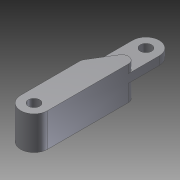
# Autodesk Inventor part: F
Saved by Autodesk Inventor 2011 SP2 (Build 150309200, 309)
## iProperties
Created: 2014-05-09
Part Number: F
Document SubType Name: Modeling
Designer: Maurice Woods
Density: 1 g/cm^3
Author: Maurice Woods
Autodesk Inventor part; units mm, degrees
ref_plane "YZ Plane" through (0, 0, 0) normal (1, 0, 0) x (0, 1, 0)
ref_plane "XZ Plane" through (0, 0, 0) normal (0, 1, 0) x (-1, 0, 0)
ref_plane "XY Plane" through (0, 0, 0) normal (0, 0, 1) x (1, 0, 0)
sketch "Sketch1" plane through (0, 0, 0) normal (0, 0, 1) x (1, 0, 0)
  line L0 (0, 20.7105) -> (0, 20.7105)
  line L1 (4, 16.7105) -> (4, 14.6095)
  line L2 (0, -20.7105) -> (0, -20.7105)
  line L3 (-4, -16.7105) -> (-4, 1.4635)
  line L4 (-4, 20.7105) -> (0, 20.7105) construction
  line L5 (0, 20.7105) -> (0, 0) construction
  line L6 (0, 0) -> (-4, 0) construction
  line L7 (-4, 0) -> (-4, 20.7105) construction
  arc A0 (4, 16.7105) -> (0, 20.7105) centre (0, 16.7105) ccw
  arc A1 (0, 20.7105) -> (-4, 16.7105) centre (0, 16.7105) ccw
  arc A2 (-4, -16.7105) -> (0, -20.7105) centre (0, -16.7105) ccw
  arc A3 (0, -20.7105) -> (4, -16.7105) centre (0, -16.7105) ccw
  line L8 (-4, 1.4635) -> (4, 14.6095)
  line L9 (-4, 1.4635) -> (-4, 16.7105)
  line L10 (4, 14.6095) -> (4, -16.7105)
  dimension "d0" = 4
  dimension "d6" = 33.421
  constraints: 22 end point, 12 tangent, 8 point on circle, 7 parallel, 4 centre point, 3 equal radius, 3 perpendicular, 2 coincident, 2 horizontal, 2 point on line, 2 other
  measures "d0" radius of A0
  measures "d6" distance of A2.centre A0.centre
extrude "Extrusion2" add sketch "Sketch1" along normal mid plane 5 contours L1 L8 L9 A1 A0
extrude "Extrusion3" add sketch "Sketch1" along normal mid plane 10 contours L10 A3 A2 L3 L8
fillet "Fillet1" radius 2 4 edges at (4, 14.6095, -3.75) (-4, 1.4635, -3.75) (4, 14.6095, 3.75) (-4, 1.4635, 3.75)
sketch "Sketch3" plane through (0, 0, -5) normal (0, 0, -1) x (-1, 0, 0)
  arc A0 (-4, -16.7105) -> (4, -16.7105) centre (0, -16.7105) ccw projected
  arc A1 (4, 16.7105) -> (-4, 16.7105) centre (0, 16.7105) ccw projected
  line L0 (-4, 7.4758) -> (-4, 16.7105) projected
  arc A2 (-0.2915, 8.5155) -> (-4, 7.4758) centre (-2, 7.4758) ccw projected
  line L1 (3.7085, 1.9425) -> (-0.2915, 8.5155) projected
  arc A3 (4, 0.9028) -> (3.7085, 1.9425) centre (2, 0.9028) ccw projected
  line L2 (4, 0.9028) -> (4, 16.7105) projected
  point P0 (0, 0)
hole "Hole2" at (0, 16.7105, -5) at (0, -16.7105, -5) direction (0, 0, 1) diameter 3.4 end through all clearance for "Socket Head Cap Screw" size "M3" standard "Ansi Metric M Profile"
sketch "Sketch4" plane through (0, 0, -2.5) normal (0, 0, -1) x (-1, 0, 0)
  circle A0 centre (0, 16.7105) radius 1.7 projected
  arc A1 (4, 16.7105) -> (-4, 16.7105) centre (0, 16.7105) ccw projected
  line L0 (-4, 7.4758) -> (-4, 16.7105) projected
  arc A2 (-0.2915, 8.5155) -> (-4, 7.4758) centre (-2, 7.4758) ccw projected
  line L1 (3.7085, 1.9425) -> (-0.2915, 8.5155) projected
  arc A3 (4, 0.9028) -> (3.7085, 1.9425) centre (2, 0.9028) ccw projected
  line L2 (4, 0.9028) -> (4, 16.7105) projected
  point P0 (0, 0)
extrude "Extrusion4" cut sketch "Sketch4" against normal up to surface (2.5 mm away)
equation "\"d6\" = LengthJ"
equation "\"LengthJ\" = 33.421041"
body "Solid2"
